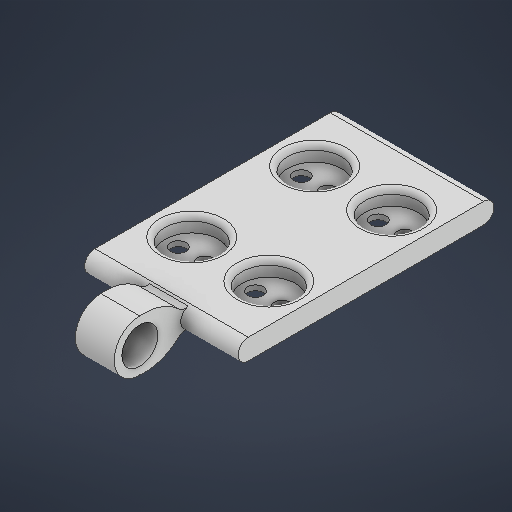
# Autodesk Inventor part: lamp_head
Saved by Autodesk Inventor 2027 (Build 310192060, 192F)
## iProperties
Created: 2026-05-15
Part Number: lamp_head
Material: Ogólny
Document SubType Name: Modeling
Designer: User
Density: 1 g/cm^3
Appearance: Domyślna
Author: User
Autodesk Inventor part; units mm, degrees
ref_plane "YZ Plane" through (0, 0, 0) normal (1, 0, 0) x (0, 1, 0)
ref_plane "XZ Plane" through (0, 0, 0) normal (0, 1, 0) x (-1, 0, 0)
sketch "Szkic1" plane through (0, 0, 0) normal (0, 1, 0) x (-1, 0, 0)
  line L0 (-7.5, 12.5) -> (7.5, 12.5)
  line L1 (7.5, 12.5) -> (7.5, -12.5)
  line L2 (7.5, -12.5) -> (-7.5, -12.5)
  line L3 (-7.5, -12.5) -> (-7.5, 12.5)
  line L4 (-7.5, 12.5) -> (7.5, -12.5) construction
  line L5 (7.5, 12.5) -> (-7.5, -12.5) construction
  line L6 (-7, 12) -> (7, 12)
  line L7 (7, 12) -> (7, -12)
  line L8 (7, -12) -> (-7, -12)
  line L9 (-7, -12) -> (-7, 12)
  line L10 (-7, 12) -> (7, -12) construction
  line L11 (7, 12) -> (-7, -12) construction
  line L12 (-2.5, 14.5) -> (2.5, 14.5)
  line L13 (2.5, 14.5) -> (2.5, 9.5)
  line L14 (2.5, 9.5) -> (-2.5, 9.5)
  line L15 (-2.5, 9.5) -> (-2.5, 14.5)
  line L16 (-2.5, 14.5) -> (2.5, 9.5) construction
  line L17 (2.5, 14.5) -> (-2.5, 9.5) construction
  line L18 (0, 12) -> (0, 8)
  circle A0 centre (0, 8) radius 2.6
  circle A1 centre (0, 0) radius 2.6
  circle A2 centre (0, -8) radius 2.6
  line L19 (0, 8) -> (-1.8, 8) construction
  line L20 (0, 8) -> (1.8, 8) construction
  circle A3 centre (-1.8, 8) radius 0.5
  circle A4 centre (1.8, 8) radius 0.5
  circle A5 centre (1.8, 0) radius 0.5
  circle A6 centre (-1.8, 0) radius 0.5
  circle A7 centre (1.8, -8) radius 0.5
  circle A8 centre (-1.8, -8) radius 0.5
  point P0 (0, 0)
  point P1 (2.5, 12)
  point P2 (-2.5, 12)
  point P3 (2.1237, 9.5)
  point P4 (-2.1237, 9.5)
  dimension "d0" = 15
  dimension "d1" = 25
  dimension "d2" = 14
  dimension "d3" = 24
  dimension "d8" = 5
  dimension "d9" = 5
  dimension "d32" = 4
  dimension "d33" = 5.2
  dimension "d36" = 8
  dimension "d41" = 1.8
  dimension "d42" = 180
  dimension "d43" = 1
  dimension "d46" = 8
  constraints: 42 end point, 9 centre point, 7 midpoint, 6 parallel, 5 horizontal, 4 perpendicular, 2 coincident, 2 vertical, 1 collinear, 1 symmetric about line, 13 other
  measures "d0" distance of L1.end L2.end
  measures "d1" distance of L0.end L1.end
  measures "d2" distance of L7.end L8.end
  measures "d3" distance of L6.end L7.end
  measures "d8" distance of L13.end L14.end
  measures "d9" distance of L12.end L13.end
  measures "d32" distance of L18.start L18.end
  measures "d33" diameter of A0
  measures "d36" distance of L19.start A1.centre
  measures "d41" distance of L19.start L19.end
  measures "d42" angle of L19 L20
  measures "d43" diameter of A3
  measures "d46" distance of A4.centre A5.centre
extrude "Wyciągnięcie proste1" add sketch "Szkic1" along normal blind 2 contours L0 L15 L6 L9 L8 L7 L13 L1 L2 L3 | L0 L13 L6 L15 | L15 L14 A0 L13 L6 L7 L8 L9 | L6 L18 A0 L14 L15 | L13 L14 A0 L18 L6 | A0 L14 L18 | L18 L14 A0 | L14 A0 | A1 | A2 | A3 | A4 | A5 | A6 | A7 | A8
extrude "Wyciągnięcie proste2" [suppressed]
ref_plane "Płaszczyzna konstrukcyjna1" through (2.5, 0, 12.5) normal (1, 0, 0) x (0, 0, -1)
sketch "Szkic2" plane through (2.5, 0, 12.5) normal (1, 0, 0) x (0, 0, -1)
  line L0 (0, 0) -> (0, 2)
  line L1 (0, 2) -> (0, 0)
  line L2 (0, 2) -> (0, 0)
  line L3 (0, 1) -> (-4, 1)
  line L4 (0, 1) -> (-4, 1) construction
  circle A0 centre (-4, 1) radius 1.75
  circle A1 centre (-4, 1) radius 2.5
  line L5 (-4, -1.5) -> (-4, -1.5)
  line L6 (-4, 3.5) -> (-4, 3.5)
  arc A2 (-4, -1.5) -> (0, 0) centre (-3.5874, 3.4829) ccw
  arc A3 (0, 2) -> (-4, 3.5) centre (-3.5874, -1.4829) ccw
  line L7 (0, 1) -> (-2.4782, 1)
  line L8 (25, 2) -> (0, 2) projected
  line L9 (25, 0) -> (0, 0) projected
  line L10 (0, 2) -> (0, 0)
  line L11 (0, 0) -> (0, 1)
  line L12 (0, 0) -> (0, 2)
  line L13 (0, 1) -> (-1.7426, 1)
  point P0 (12.5, 0)
  point P1 (-4, -1.5)
  dimension "d11" = 4
  dimension "d12" = 0
  dimension "d13" = 3.5
  dimension "d14" = 5
  dimension "d15" = 0
  dimension "d16" = 0
  dimension "d17" = 5
  dimension "d18" = 5
  constraints: 24 end point, 6 point on circle, 4 centre point, 3 midpoint, 2 coincident, 2 horizontal, 2 perpendicular, 1 collinear, 1 vertical
  measures "d11" distance of L3.start L3.end
  measures "d12" distance between parallel lines of L3 L4
  measures "d13" diameter of A0
  measures "d14" diameter of A1
  measures "d15" distance of L5.start L5.end
  measures "d16" distance of L6.start L6.end
  measures "d17" radius of A2
  measures "d18" radius of A3
extrude "Wyciągnięcie proste3" add sketch "Szkic2" along normal mid plane 3.8
fillet "Zaokrąglenie1" radius 1 4 edges at (5.95, 2, 12.5) (5.95, 0, 12.5) (-3.45, 2, 12.5) (-3.45, 0, 12.5)
fillet "Zaokrąglenie2" radius 1 2 edges at (0, 2, -12.5) (0, 0, -12.5)
fillet "Zaokrąglenie3" radius 1 6 edges at (1.25, 1.6904, 12.2234) (2.5, 1.6904, 12.2234) (3.75, 1.6904, 12.2234) (1.25, 0.3096, 12.2234) (2.5, 0.3096, 12.2234) (3.75, 0.3096, 12.2234)
ref_plane "Płaszczyzna konstrukcyjna3" through (0, 0, -9) normal (0, 0, 1) x (1, 0, 0)
move faces "Przesuń1" translate (-2.5, 0, 0) faces at (0.6, 0.0919, 12.277) (0.6, 1.9081, 12.277) (0.6, 0.2429, 12.4444) (0.6, 1.7571, 12.4444) (0.6, 0.4621, 13.3337) (4.4, 0.0919, 12.277) (4.4, 0.2429, 12.4444) (4.4, 1.7571, 12.4444) (4.4, 1.9081, 12.277) (4.4, 0.4621, 13.3337)
sketch "Szkic6" plane through (0, 2, 0) normal (0, 1, 0) x (1, 0, 0)
  line L0 (7.5, -11.5) -> (7.5, 11.5) projected
  line L1 (7.5, -11.5) -> (0, 0) construction
  line L2 (7.5, 0) -> (0, -11.5) construction
  line L3 (7.5356, 0.0547) -> (-7.5, 0) construction
  line L4 (-7.5, 11.5) -> (-7.5, -11.5) projected
  line L5 (0, -11.5) -> (0, 11.5) construction
  line L6 (7.5, 11.5) -> (-7.5, 11.5) projected
  circle A0 centre (3.75, -5.75) radius 2.6
  line L7 (3.75, -5.75) -> (6.35, -5.75)
  line L8 (3.75, -5.75) -> (1.15, -5.75)
  circle A1 centre (5.05, -5.75) radius 0.75
  circle A2 centre (2.45, -5.75) radius 0.75
  circle A3 centre (-3.75, -5.7773) radius 2.6
  circle A4 centre (-5.05, -5.7773) radius 0.75
  circle A5 centre (-2.45, -5.7773) radius 0.75
  circle A6 centre (3.75, 6.25) radius 2.6
  circle A7 centre (2.45, 6.25) radius 0.75
  circle A8 centre (5.05, 6.25) radius 0.75
  circle A9 centre (-3.75, 6.2227) radius 2.6
  circle A10 centre (-5.05, 6.2227) radius 0.75
  circle A11 centre (-2.45, 6.2227) radius 0.75
  point P0 (-1.15, -5.7773)
  point P1 (-6.35, -5.7773)
  point P2 (6.35, 6.25)
  point P3 (1.15, 6.25)
  point P4 (-1.15, 6.2227)
  point P5 (-6.35, 6.2227)
  dimension "d23" = 1
  dimension "d65" = 5.2
  dimension "d66" = 1.5
  dimension "d67" = 1.5
  dimension "d70" = 7.5
  dimension "d73" = 12
  constraints: 12 centre point, 12 end point, 8 point on circle, 6 midpoint, 2 point on line, 1 vertical, 25 other
  measures "d65" diameter of A0
  measures "d66" diameter of A1
  measures "d67" diameter of A2
  measures "d70" distance of L7.start A3.centre
  measures "d73" distance of L7.start A6.centre
extrude "Wyciągnięcie proste6" cut sketch "Szkic6" against normal blind 1.5 contours L7 A1 L8 A2 A0 | A0 L8 A2 L7 A1 | A3 | A6 | A9
extrude "Wyciągnięcie proste7" cut sketch "Szkic6" against normal blind 5.2 contours A1 L7 | L7 A1 | A2 L8 | L8 A2 | A4 | A5 | A7 | A8 | A10 | A11
fillet "Zaokrąglenie5" radius 0.5 4 edges at (1.15, 2, -6.25) (1.15, 2, 5.75) (-6.35, 2, 5.7773) (-6.35, 2, -6.2227)
equation "\"d78\" = d65"
